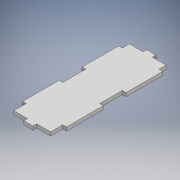
# Autodesk Inventor part: F7
Saved by Autodesk Inventor 2018 (Build 220112000, 112)
## iProperties
Created: 2018-03-06
Part Number: F7
Material: Generic
Document SubType Name: Modeling
Designer: isai
Density: 1 g/cm^3
Appearance: Default
Author: isai
Autodesk Inventor part; units mm, degrees
ref_plane "YZ Plane" through (0, 0, 0) normal (1, 0, 0) x (0, 1, 0)
ref_plane "XZ Plane" through (0, 0, 0) normal (0, 1, 0) x (-1, 0, 0)
sketch "Sketch1" plane through (0, 0, 0) normal (0, 0, 1) x (1, 0, 0)
  line L0 (-101, -200.839) -> (-97, -200.839)
  line L1 (-97, -200.839) -> (-97, -240.839)
  line L2 (-97, -240.839) -> (-101, -240.839)
  line L3 (-101, -240.839) -> (-101, -258.2)
  line L4 (-101, -128.2) -> (-101, -135.9372)
  line L5 (-101, -135.9372) -> (-97, -135.9372)
  line L6 (-97, -135.9372) -> (-97, -175.9372)
  line L7 (-97, -175.9372) -> (-101, -175.9372)
  line L8 (-101, -175.9372) -> (-101, -200.839)
  line L9 (-101, -258.2) -> (-101, -254.2)
  line L10 (-101, -254.2) -> (-141, -254.2)
  line L11 (-101, -128.2) -> (-141, -128.2)
  line L12 (-121, -128.2) -> (-121, -103.1789)
  line L13 (-145, -200.839) -> (-145, -240.839)
  line L14 (-145, -240.839) -> (-141, -240.839)
  line L15 (-141, -200.839) -> (-145, -200.839)
  line L16 (-145, -175.9372) -> (-141, -175.9372)
  line L17 (-145, -135.9372) -> (-145, -175.9372)
  line L18 (-141, -135.9372) -> (-145, -135.9372)
  line L19 (-141, -135.9372) -> (-141, -128.2)
  line L20 (-141, -254.2) -> (-141, -240.839)
  line L21 (-141, -200.839) -> (-141, -175.9372)
  point P0 (0, 0)
  dimension "d0" = 4
  dimension "d1" = 40
  dimension "d2" = 40
  dimension "d3" = 40
  constraints: 44 end point, 8 symmetric about line, 4 perpendicular, 1 horizontal, 1 midpoint, 1 point on line, 1 vertical
  measures "d0" distance of L3.end L9.end
  measures "d1" distance of L9.end L10.end
  measures "d2" distance of L6.start L7.start
  measures "d3" distance of L1.start L1.end
extrude "Extrusion1" add sketch "Sketch1" along normal blind 4
sketch "Sketch2" plane through (0, 0, 4) normal (0, 0, 1) x (1, 0, 0)
  line L0 (-97, -200.839) -> (-101, -200.839) projected
  line L1 (-101, -200.839) -> (-101, -175.9372) projected
  line L2 (-101, -175.9372) -> (-97, -175.9372) projected
  line L3 (-97, -175.9372) -> (-97, -135.9372) projected
  line L4 (-97, -135.9372) -> (-101, -135.9372) projected
  line L5 (-101, -135.9372) -> (-101, -128.2) projected
  line L6 (-101, -128.2) -> (-141, -128.2) projected
  line L7 (-141, -128.2) -> (-141, -135.9372) projected
  line L8 (-141, -135.9372) -> (-145, -135.9372) projected
  line L9 (-145, -135.9372) -> (-145, -175.9372) projected
  line L10 (-145, -175.9372) -> (-141, -175.9372) projected
  line L11 (-141, -175.9372) -> (-141, -200.839) projected
  line L12 (-141, -200.839) -> (-145, -200.839) projected
  line L13 (-145, -200.839) -> (-145, -240.839) projected
  line L14 (-145, -240.839) -> (-141, -240.839) projected
  line L15 (-141, -240.839) -> (-141, -254.2) projected
  line L16 (-141, -254.2) -> (-101, -254.2) projected
  line L17 (-101, -254.2) -> (-101, -240.839) projected
  line L18 (-101, -240.839) -> (-97, -240.839) projected
  line L19 (-97, -240.839) -> (-97, -200.839) projected
  line L20 (-126, -128.2) -> (-116, -128.2)
  line L21 (-116, -128.2) -> (-116, -124.2)
  line L22 (-116, -124.2) -> (-126, -124.2)
  line L23 (-126, -124.2) -> (-126, -128.2)
  point P0 (0, 0)
  point P1 (-121, -128.2)
  dimension "d6" = 10
  dimension "d7" = 4
  constraints: 8 end point, 2 midpoint, 2 parallel, 1 horizontal, 1 perpendicular
  measures "d6" distance of L22.end L21.end
  measures "d7" distance of L21.end L20.end
extrude "Extrusion2" add sketch "Sketch2" against normal blind 4 contours L6 L23 L22 L21
ref_plane "Work Plane1" through (-101, -191.2, 4) normal (0, 1, 0) x (1, 0, 0)
mirror "Mirror1" about plane through (-101, -191.2, 4) normal (0, 1, 0) of "Extrusion2"
body "Solid1"
